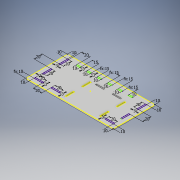
# Autodesk Inventor part: base
Saved by Autodesk Inventor 2017.2 (Build 212233000, 233)
## iProperties
Created: 2017-06-02
Part Number: base
Material: Generic
Document SubType Name: Modeling
Designer: SandeepSH
Density: 1 g/cm^3
Appearance: Default
Author: SandeepSH
Autodesk Inventor part; units mm, degrees
ref_plane "YZ Plane" through (0, 0, 0) normal (1, 0, 0) x (0, 1, 0)
ref_plane "XZ Plane" through (0, 0, 0) normal (0, 1, 0) x (-1, 0, 0)
ref_plane "XY Plane" through (0, 0, 0) normal (0, 0, 1) x (1, 0, 0)
sketch "Sketch1" plane through (0, 0, 0) normal (0, 1, 0) x (-1, 0, 0)
  point P0 (0, 0)
sketch "Sketch2" plane through (0, 0, 0) normal (0, 1, 0) x (-1, 0, 0)
  line L0 (105, 50) -> (-105, 50)
  line L1 (-105, 50) -> (-105, -50)
  line L2 (-105, -50) -> (105, -50)
  line L3 (105, -50) -> (105, 50)
  line L4 (105, 50) -> (-105, -50) construction
  line L5 (-105, 50) -> (105, -50) construction
  point P0 (0, 0)
  dimension "d0" = 210
  dimension "d1" = 100
  constraints: 12 end point, 2 midpoint, 2 parallel, 1 horizontal, 1 perpendicular
  measures "d0" distance of L2.end L1.end
  measures "d1" distance of L1.end L0.end
extrude "Extrusion1" add sketch "Sketch2" along normal blind 3
sketch "Sketch3" plane through (0, 3, 0) normal (0, 1, 0) x (1, 0, 0)
  line L0 (-21, 0) -> (-18, 0)
  line L1 (-18, 0) -> (-18, 20)
  line L2 (-18, 20) -> (-21, 20)
  line L3 (-21, 20) -> (-21, 0)
  line L4 (-21, 0) -> (-18, 20) construction
  line L5 (-18, 0) -> (-21, 20) construction
  line L6 (105, 50) -> (-105, 50) projected
  line L7 (62, 20) -> (65, 20)
  line L8 (65, 20) -> (65, 0)
  line L9 (65, 0) -> (62, 0)
  line L10 (62, 0) -> (62, 20)
  line L11 (62, 20) -> (65, 0) construction
  line L12 (65, 20) -> (62, 0) construction
  line L13 (105, -50) -> (105, 50) projected
  line L14 (-21, -40) -> (-18, -40)
  line L15 (-18, -40) -> (-18, -20)
  line L16 (-18, -20) -> (-21, -20)
  line L17 (-21, -20) -> (-21, -40)
  line L18 (-21, -40) -> (-18, -20) construction
  line L19 (-18, -40) -> (-21, -20) construction
  line L20 (-105, -50) -> (105, -50) projected
  line L21 (62, -20) -> (65, -20)
  line L22 (65, -20) -> (65, -40)
  line L23 (65, -40) -> (62, -40)
  line L24 (62, -40) -> (62, -20)
  line L25 (62, -20) -> (65, -40) construction
  line L26 (65, -20) -> (62, -40) construction
  line L27 (-8, 24.65) -> (12, 24.65)
  line L28 (12, 24.65) -> (12, 21.65)
  line L29 (12, 21.65) -> (-8, 21.65)
  line L30 (-8, 21.65) -> (-8, 24.65)
  line L31 (-8, 24.65) -> (12, 21.65) construction
  line L32 (12, 24.65) -> (-8, 21.65) construction
  line L33 (32, 24.65) -> (52, 24.65)
  line L34 (52, 24.65) -> (52, 21.65)
  line L35 (52, 21.65) -> (32, 21.65)
  line L36 (32, 21.65) -> (32, 24.65)
  line L37 (32, 24.65) -> (52, 21.65) construction
  line L38 (52, 24.65) -> (32, 21.65) construction
  line L39 (-105, -50) -> (105, -50) projected
  line L40 (105, -50) -> (105, 50) projected
  line L41 (105, 50) -> (-105, 50) projected
  line L42 (-105, 50) -> (-105, -50) projected
  point P0 (0, 0)
  point P1 (-19.5, 10)
  point P2 (63.5, 10)
  point P3 (-19.5, -30)
  point P4 (63.5, -30)
  point P5 (2, 23.15)
  point P6 (42, 23.15)
  dimension "d4" = 3
  dimension "d5" = 20
  dimension "d6" = 30
  dimension "d7" = 3
  dimension "d8" = 20
  dimension "d9" = 30
  dimension "d10" = 80
  dimension "d11" = 40
  dimension "d14" = 20
  dimension "d15" = 10
  dimension "d16" = 20
  dimension "d17" = 3
  dimension "d18" = 10
  dimension "d19" = 20
  dimension "d20" = 3
  dimension "d21" = 10
  constraints: 72 end point, 12 midpoint, 12 parallel, 6 horizontal, 6 perpendicular, 2 collinear
  measures "d4" distance of L2.end L1.end
  measures "d5" distance of L1.end L0.end
  measures "d6" distance between parallel lines of L6 L2
  measures "d7" distance of L8.end L9.end
  measures "d8" distance of L7.end L8.end
  measures "d9" distance between parallel lines of L7 L6
  measures "d10" distance between parallel lines of L10 L1
  measures "d11" distance between parallel lines of L13 L8
  measures "d14" distance of L15.end L14.end
  measures "d15" distance between parallel lines of L20 L14
  measures "d16" distance of L28.end L29.end
  measures "d17" distance of L27.end L28.end
  measures "d18" distance between parallel lines of L30 L1
  measures "d19" distance of L34.end L35.end
  measures "d20" distance of L33.end L34.end
  measures "d21" distance from line of L10 L33.end
extrude "Extrusion2" cut sketch "Sketch3" against normal through all contours L3 L2 L1 L0 | L7 L8 L9 L10
sketch "Sketch4" plane through (0, 3, 0) normal (0, 1, 0) x (1, 0, 0)
  point P0 (0, 0)
sketch "Sketch5" plane through (0, 3, 0) normal (0, 1, 0) x (1, 0, 0)
  line L0 (-21, 0) -> (-21, 20) projected
  line L1 (-18, 20) -> (-18, 0) projected
  line L2 (-21, 20) -> (-18, 20) projected
  line L3 (-18, 0) -> (-21, 0) projected
  line L4 (62, 0) -> (62, 20) projected
  line L5 (65, 0) -> (62, 0) projected
  line L6 (65, 20) -> (65, 0) projected
  line L7 (62, 20) -> (65, 20) projected
  point P0 (0, 0)
sketch "Sketch6" plane through (0, 3, 0) normal (0, 1, 0) x (1, 0, 0)
  line L0 (-21, 0) -> (-18, 0)
  line L1 (-18, 0) -> (-18, 20)
  line L2 (-18, 20) -> (-21, 20)
  line L3 (-21, 20) -> (-21, 0)
  line L4 (-21, 0) -> (-18, 20) construction
  line L5 (-18, 0) -> (-21, 20) construction
  line L6 (105, 50) -> (-105, 50)
  line L7 (62, 20) -> (65, 20)
  line L8 (65, 20) -> (65, 0)
  line L9 (65, 0) -> (62, 0)
  line L10 (62, 0) -> (62, 20)
  line L11 (62, 20) -> (65, 0) construction
  line L12 (65, 20) -> (62, 0) construction
  line L13 (105, -50) -> (105, 50)
  line L14 (-21, -40) -> (-18, -40)
  line L15 (-18, -40) -> (-18, -20)
  line L16 (-18, -20) -> (-21, -20)
  line L17 (-21, -20) -> (-21, -40)
  line L18 (-21, -40) -> (-18, -20) construction
  line L19 (-18, -40) -> (-21, -20) construction
  line L20 (-105, -50) -> (105, -50)
  line L21 (62, -20) -> (65, -20)
  line L22 (65, -20) -> (65, -40)
  line L23 (65, -40) -> (62, -40)
  line L24 (62, -40) -> (62, -20)
  line L25 (62, -20) -> (65, -40) construction
  line L26 (65, -20) -> (62, -40) construction
  line L27 (-8, 23) -> (12, 23)
  line L28 (12, 23) -> (12, 20)
  line L29 (12, 20) -> (-8, 20)
  line L30 (-8, 20) -> (-8, 23)
  line L31 (-8, 23) -> (12, 20) construction
  line L32 (12, 23) -> (-8, 20) construction
  line L33 (32, 23) -> (52, 23)
  line L34 (52, 23) -> (52, 20)
  line L35 (52, 20) -> (32, 20)
  line L36 (32, 20) -> (32, 23)
  line L37 (32, 23) -> (52, 20) construction
  line L38 (52, 23) -> (32, 20) construction
  line L39 (-105, -50) -> (105, -50)
  line L40 (105, -50) -> (105, 50)
  line L41 (105, 50) -> (-105, 50)
  line L42 (-105, 50) -> (-105, -50)
  point P0 (0, 0)
  point P1 (0, 0)
  point P2 (-19.5, 10)
  point P3 (63.5, 10)
  point P4 (-19.5, -30)
  point P5 (63.5, -30)
  point P6 (2, 21.5)
  point P7 (42, 21.5)
  dimension "d22" = 3
  dimension "d23" = 20
  dimension "d24" = 30
  dimension "d25" = 3
  dimension "d26" = 20
  dimension "d27" = 30
  dimension "d28" = 80
  dimension "d29" = 40
  dimension "d30" = 20
  dimension "d31" = 10
  dimension "d32" = 20
  dimension "d33" = 3
  dimension "d34" = 10
  dimension "d35" = 20
  dimension "d36" = 3
  dimension "d37" = 10
  dimension "d41" = 100
  dimension "d42" = 70
  constraints: 86 end point, 12 midpoint, 12 parallel, 6 horizontal, 6 perpendicular, 3 collinear
  measures "d22" distance of L2.end L1.end
  measures "d23" distance of L1.end L0.end
  measures "d24" distance between parallel lines of L6 L2
  measures "d25" distance of L8.end L9.end
  measures "d26" distance of L7.end L8.end
  measures "d27" distance between parallel lines of L7 L6
  measures "d28" distance between parallel lines of L10 L1
  measures "d29" distance between parallel lines of L13 L8
  measures "d30" distance of L15.end L14.end
  measures "d31" distance between parallel lines of L20 L14
  measures "d32" distance of L28.end L29.end
  measures "d33" distance of L27.end L28.end
  measures "d34" distance between parallel lines of L30 L1
  measures "d35" distance of L34.end L35.end
  measures "d36" distance of L33.end L34.end
  measures "d37" distance from line of L10 L33.end
  measures "d41" distance between parallel lines of L20 L6
  measures "d42" distance between parallel lines of L20 L29
extrude "Extrusion3" cut sketch "Sketch6" against normal through all contours L17 L16 L15 L14 | L21 L22 L23 L24 | L27 L28 L29 L30 | L33 L34 L35 L36
fillet "Fillet1" radius 2 4 edges at (-105, 1.5, 50) (105, 1.5, 50) (105, 1.5, -50) (-105, 1.5, -50)
sketch "Sketch7" plane through (0, 3, 0) normal (0, 1, 0) x (1, 0, 0)
  line L0 (-21, -40) -> (-21, -20) projected
  line L1 (-18, -20) -> (-18, -40) projected
  line L2 (-21, -20) -> (-18, -20) projected
  line L3 (-18, -40) -> (-21, -40) projected
  line L4 (62, -40) -> (62, -20) projected
  line L5 (65, -40) -> (62, -40) projected
  line L6 (65, -20) -> (65, -40) projected
  line L7 (62, -20) -> (65, -20) projected
  line L8 (-105, 48) -> (-105, -48) projected
  line L9 (-103, -50) -> (103, -50) projected
  line L10 (-95, -40) -> (-75, -40)
  line L11 (-75, -40) -> (-75, -37)
  line L12 (-75, -37) -> (-95, -37)
  line L13 (-95, -37) -> (-95, -40)
  line L14 (-55, -40) -> (-35, -40)
  line L15 (-35, -40) -> (-35, -37)
  line L16 (-35, -37) -> (-55, -37)
  line L17 (-55, -37) -> (-55, -40)
  line L18 (105, -48) -> (105, 48) projected
  line L19 (95, -40) -> (75, -40)
  line L20 (75, -40) -> (75, -37)
  line L21 (75, -37) -> (95, -37)
  line L22 (95, -37) -> (95, -40)
  line L23 (103, 50) -> (-103, 50) projected
  line L24 (-95, 40) -> (-92, 40)
  line L25 (-92, 40) -> (-92, 20)
  line L26 (-92, 20) -> (-95, 20)
  line L27 (-95, 20) -> (-95, 40)
  line L28 (-95, 0) -> (-92, 0)
  line L29 (-92, 0) -> (-92, -20)
  line L30 (-92, -20) -> (-95, -20)
  line L31 (-95, -20) -> (-95, 0)
  line L32 (95, 40) -> (92, 40)
  line L33 (92, 40) -> (92, 20)
  line L34 (92, 20) -> (95, 20)
  line L35 (95, 20) -> (95, 40)
  line L36 (95, -20) -> (92, -20)
  line L37 (92, -20) -> (92, 0)
  line L38 (92, 0) -> (95, 0)
  line L39 (95, 0) -> (95, -20)
  line L40 (-72, 40) -> (-62, 40)
  line L41 (-62, 40) -> (-62, 37)
  line L42 (-62, 37) -> (-72, 37)
  line L43 (-72, 37) -> (-72, 40)
  line L44 (-47, 40) -> (-37, 40)
  line L45 (-37, 40) -> (-37, 37)
  line L46 (-37, 37) -> (-47, 37)
  line L47 (-47, 37) -> (-47, 40)
  line L48 (-22, 40) -> (-12, 40)
  line L49 (-12, 40) -> (-12, 37)
  line L50 (-12, 37) -> (-22, 37)
  line L51 (-22, 37) -> (-22, 40)
  line L52 (3, 40) -> (13, 40)
  line L53 (13, 40) -> (13, 37)
  line L54 (13, 37) -> (3, 37)
  line L55 (3, 37) -> (3, 40)
  line L56 (28, 40) -> (38, 40)
  line L57 (38, 40) -> (38, 37)
  line L58 (38, 37) -> (28, 37)
  line L59 (28, 37) -> (28, 40)
  line L60 (53, 37) -> (63, 37)
  line L61 (63, 37) -> (63, 40)
  line L62 (63, 40) -> (53, 40)
  line L63 (53, 40) -> (53, 37)
  point P0 (0, 0)
  dimension "d43" = 10
  dimension "d44" = 10
  dimension "d45" = 20
  dimension "d46" = 3
  dimension "d47" = 20
  dimension "d48" = 3
  dimension "d49" = 20
  dimension "d50" = 10
  dimension "d51" = 10
  dimension "d52" = 20
  dimension "d53" = 3
  dimension "d54" = 10
  dimension "d55" = 10
  dimension "d56" = 10
  dimension "d57" = 10
  dimension "d58" = 3
  dimension "d59" = 20
  dimension "d60" = 3
  dimension "d61" = 20
  dimension "d62" = 20
  dimension "d63" = 3
  dimension "d64" = 20
  dimension "d65" = 20
  dimension "d66" = 10
  dimension "d67" = 3
  dimension "d68" = 20
  dimension "d69" = 10
  dimension "d70" = 3
  dimension "d71" = 15
  dimension "d72" = 10
  dimension "d73" = 10
  dimension "d74" = 10
  dimension "d75" = 15
  dimension "d76" = 15
  dimension "d77" = 15
  dimension "d78" = 10
  dimension "d79" = 15
  constraints: 104 end point, 26 parallel, 13 horizontal, 13 perpendicular, 8 point on line
  measures "d43" distance from line of L8 L10.start
  measures "d44" distance from line of L9 L10.start
  measures "d45" distance of L12.end L11.end
  measures "d46" distance of L11.end L10.end
  measures "d47" distance of L16.end L15.end
  measures "d48" distance of L15.end L14.end
  measures "d49" distance between parallel lines of L11 L17
  measures "d50" distance from line of L9 L19.start
  measures "d51" distance from line of L19.start L18
  measures "d52" distance of L20.end L21.end
  measures "d53" distance of L19.end L20.end
  measures "d54" distance from line of L23 L24.start
  measures "d55" distance from line of L8 L24.start
  measures "d56" distance from line of L18 L32.start
  measures "d57" distance from line of L23 L32.start
  measures "d58" distance of L25.end L26.end
  measures "d59" distance of L24.end L25.end
  measures "d60" distance of L29.end L30.end
  measures "d61" distance of L28.end L29.end
  measures "d62" distance between parallel lines of L28 L26
  measures "d63" distance of L34.end L33.end
  measures "d64" distance of L33.end L32.end
  measures "d65" distance between parallel lines of L38 L34
  measures "d66" distance of L41.end L42.end
  measures "d67" distance of L40.end L41.end
  measures "d68" distance between parallel lines of L43 L25
  measures "d69" distance of L45.end L46.end
  measures "d70" distance of L44.end L45.end
  measures "d71" distance between parallel lines of L47 L41
  measures "d72" distance of L49.end L50.end
  measures "d73" distance of L53.end L54.end
  measures "d74" distance of L57.end L58.end
  measures "d75" distance between parallel lines of L51 L45
  measures "d76" distance between parallel lines of L55 L49
  measures "d77" distance between parallel lines of L59 L53
  measures "d78" distance of L62.end L61.end
  measures "d79" distance between parallel lines of L63 L57
equation "\"d9\" = d6"
equation "\"d21\" = d18"
equation "\"d27\" = d24"
equation "\"d37\" = d34"
equation "\"d44\" = d43"
equation "\"d75\" = d71"
equation "\"d76\" = d75"
equation "\"d77\" = d76"
equation "\"d79\" = d76"
body "Solid1"
